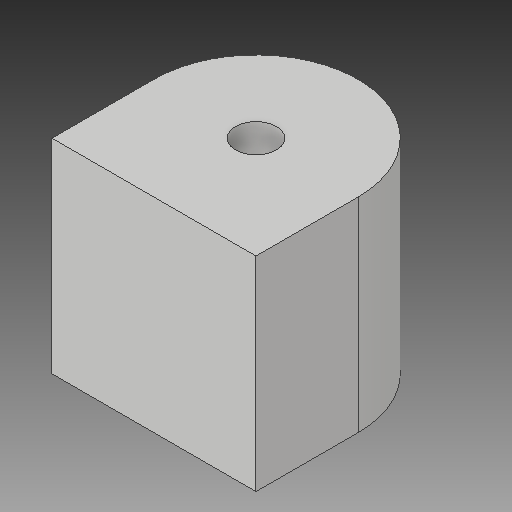
# Autodesk Inventor part: Hinge
Saved by Autodesk Inventor 2019 (Build 230136000, 136)
## iProperties
Created: 2019-09-29
Part Number: Hinge
Material: Generic
Document SubType Name: Modeling
Designer: james
Density: 1 g/cm^3
Appearance: Default
Mass: 14.1139 g
Surface Area: 38.2043 cm^2
Volume: 14.1139 cm^3
Author: james
Autodesk Inventor part; units mm, degrees
ref_plane "YZ Plane" through (0, 0, 0) normal (1, 0, 0) x (0, 1, 0)
ref_plane "XZ Plane" through (0, 0, 0) normal (0, 1, 0) x (-1, 0, 0)
ref_plane "XY Plane" through (0, 0, 0) normal (0, 0, 1) x (1, 0, 0)
sketch "Sketch1" plane through (0, 0, 0) normal (0, 1, 0) x (-1, 0, 0)
  line L0 (11.3393, 25.914) -> (-14.0607, 25.914)
  line L1 (-14.0607, 25.914) -> (-14.0607, 13.214)
  line L2 (11.3393, 13.214) -> (11.3393, 25.914)
  arc A0 (-14.0607, 13.214) -> (11.3393, 13.214) centre (-1.3607, 13.214) ccw
  point P0 (0, 0)
  dimension "d1" = 25.4
  dimension "d2" = 25.4
  dimension "d3" = 12.7
  dimension "d4" = 12.7
  constraints: 6 end point, 2 point on circle, 1 centre point, 1 horizontal, 1 parallel, 1 perpendicular
  measures "d1" distance of L0.start L0.end
  measures "d2" diameter of A0
  measures "d3" distance from line of L0 A0.centre
  measures "d4" distance from line of L2 A0.centre
extrude "Extrusion1" add sketch "Sketch1" along normal blind 25.4
sketch "Sketch2" plane through (0, 25.4, 0) normal (0, 1, 0) x (1, 0, 0)
  arc A0 (14.0607, -13.214) -> (-11.3393, -13.214) centre (1.3607, -13.214) ccw projected
  circle A1 centre (1.3607, -13.214) radius 2.54
  point P0 (0, 0)
  dimension "d7" = 5.08
  constraints: 1 centre point, 1 coincident
  measures "d7" diameter of A1
extrude "Extrusion2" cut sketch "Sketch2" against normal blind 25.4
body "Solid1"
